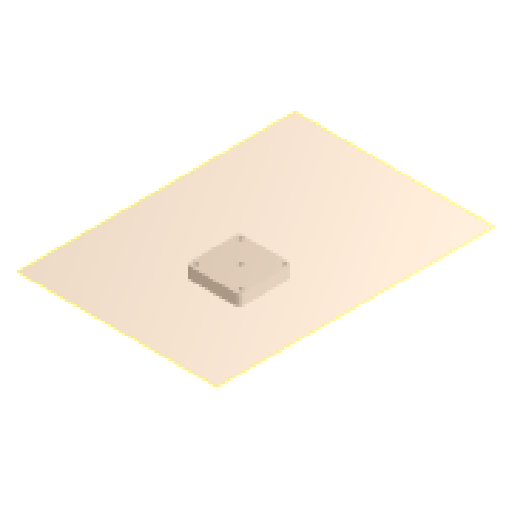
# Autodesk Inventor part: 00_Micro_Stepper_15mm_Gearbox_counterbearing
Saved by Autodesk Inventor 2024.1 (Build 281209000, 209)
## iProperties
Created: 2024-08-30
Part Number: 00_Micro_Stepper_15mm_Gearbox_counterbearing
Material: Generisch
Document SubType Name: Modeling
Designer: diederichbenedict
Density: 1 g/cm^3
Appearance: Vorgabe
Author: diederichbenedict
Autodesk Inventor part; units mm, degrees
ref_plane "YZ Plane" through (0, 0, 0) normal (1, 0, 0) x (0, 1, 0)
ref_plane "XZ Plane" through (0, 0, 0) normal (0, 1, 0) x (-1, 0, 0)
ref_plane "XY Plane" through (0, 0, 0) normal (0, 0, 1) x (1, 0, 0)
ref_plane "Arbeitsebene1" through (0, 0, 0) normal (0, 0, 1) x (1, 0, 0)
sketch "Skizze1" plane through (0, 0, 0) normal (0, 0, 1) x (1, 0, 0)
  line L0 (11.7109, -4.9124) -> (9.211, -4.9293) projected
  line L1 (9.211, -4.9293) -> (9.1974, -2.9294) projected
  line L2 (9.1974, -2.9294) -> (-3.8023, -3.0177) projected
  line L3 (-3.8023, -3.0177) -> (-3.8306, 1.1495) projected
  line L4 (-3.8306, 1.1495) -> (-6.8306, 1.1291) projected
  line L5 (-6.8306, 1.1291) -> (-6.6653, -23.2049) projected
  line L6 (-6.6653, -23.2049) -> (-3.6653, -23.1845) projected
  line L7 (-3.6653, -23.1845) -> (-3.6937, -19.0173) projected
  line L8 (-3.6937, -19.0173) -> (9.306, -18.929) projected
  line L9 (9.306, -18.929) -> (9.2925, -16.9291) projected
  line L10 (9.2925, -16.9291) -> (11.7924, -16.9121) projected
  line L11 (11.7924, -16.9121) -> (11.7109, -4.9124) projected
  circle A0 centre (13.7364, 0.5156) radius 1.025 projected
  circle A1 centre (13.7676, -22.4844) radius 1.025 projected
  circle A2 centre (-9.2323, -22.5156) radius 1.025 projected
  circle A3 centre (-9.2636, 0.4844) radius 1.025 projected
  line L12 (-11.8291, 0.9046) -> (-11.6661, -23.0948) projected
  arc A4 (-9.8428, 2.9182) -> (-11.8291, 0.9046) centre (-9.8292, 0.9182) ccw projected
  line L13 (14.1567, 3.0812) -> (-9.8428, 2.9182) projected
  arc A5 (16.1702, 1.0948) -> (14.1567, 3.0812) centre (14.1703, 1.0812) ccw projected
  line L14 (16.3332, -22.9046) -> (16.1702, 1.0948) projected
  arc A6 (14.3468, -24.9182) -> (16.3332, -22.9046) centre (14.3333, -22.9182) ccw projected
  line L15 (-9.6526, -25.0812) -> (14.3468, -24.9182) projected
  arc A7 (-11.6661, -23.0948) -> (-9.6526, -25.0812) centre (-9.6662, -23.0812) ccw projected
  circle A8 centre (2.252, -11) radius 7.5 projected
  circle A9 centre (2.252, -11) radius 1.5
  circle A10 centre (-9.2323, -22.5156) radius 1.4
  circle A11 centre (13.7676, -22.4844) radius 1.4
  circle A12 centre (-9.2636, 0.4844) radius 1.4
  circle A13 centre (13.7364, 0.5156) radius 1.4
  point P0 (0, 0)
  dimension "d0" = 3
  dimension "d1" = 2.8
  dimension "d2" = 2.8
  dimension "d3" = 2.8
  dimension "d4" = 2.8
  constraints: 5 centre point, 5 coincident
  measures "d0" diameter of A9
  measures "d1" diameter of A10
  measures "d2" diameter of A11
  measures "d3" diameter of A12
  measures "d4" diameter of A13
extrude "Extrusion1" add sketch "Skizze1" against normal blind 6 contours L11 L10 L9 L8 L7 L6 L5 L4 L3 L2 L1 L0 | A4 L13 A5 L14 A6 L15 A7 L12 | A8
